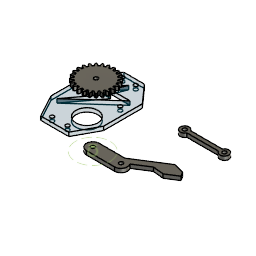
ARM (Autodesk Fusion 360 archive; units mm, degrees)
design "Untitled"
part number: 2026-04-05-15-25-42-375
Autodesk Fusion 360 part; units mm, degrees
note: some values were not read from the file. Chosen so that the rebuilt part matches the saved one: that a step has no effect. Set by a fixed rule: which sketch regions a step uses.
sketch "Sketch1" plane through (0, 0, 0) normal (0, 0, 1) x (1, 0, 0)
  line L0 (0, -5) -> (22, -5)
  arc A0 (22, -5) -> (22, 5) centre (22, 0) ccw
  line L1 (22, 5) -> (0, 5)
  arc A1 (0, 5) -> (0, -5) centre (0, 0) ccw
  line L2 (0, 0) -> (22, 0) construction
  line L3 (20.05, 5) -> (48.773, 23.1931)
  line L4 (48.773, 23.1931) -> (56.2338, 11.4141)
  line L5 (25.5276, -3.5434) -> (54.2034, 14.6197)
  line L6 (44.0321, 20.1901) -> (52.5034, 17.9377)
  line L7 (45.5663, 9.149) -> (37.2965, 10.0791)
  line L8 (37.2965, 10.0791) -> (26.0383, 2.9482)
  circle A2 centre (0, 0) radius 1.5
  circle A3 centre (22, 0) radius 1.5
  dimension "d1" = 22
  dimension "d2" = 5
  dimension "d3" = 147.65
  dimension "d4" = 34
  dimension "d6" = 1.95
  dimension "d7" = 3
  dimension "d8" = 3
  constraint tangent L0 A0
  constraint tangent A0 L1
  constraint parallel L0 L1
  constraint tangent L1 A1
  constraint tangent L0 A1
  constraint horizontal L2
  constraint coincident A1.centre L2.start
  constraint coincident L1 L3.start
  constraint perpendicular L3 L4
  constraint coincident A0 L5.start
  constraint coincident L4 L5.end
  constraint perpendicular L4 L5
  constraint coincident L3 L6.start
  constraint coincident L5 L7.start
  constraint coincident A0 L8.end
  constraint parallel L5 L8
  constraint concentric A1 A2
  constraint concentric A0 A3
  measures "d1" distance of A1.centre A0.centre
  measures "d2" radius of A1
  measures "d3" angle of L1 L3
  measures "d4" distance of L3.start L3.end
  measures "d6" horizontal distance of A0.centre L3.start
  measures "d7" diameter of A2
  measures "d8" diameter of A3
extrude "Extrude1" add sketch "Sketch1" along normal blind 3 contours L0 A0 L1 A1 | A0 L1 L3 L4 L5 L6 L7 L8 makes body 1
sketch "Sketch2" plane through (0, 0, 0) normal (0, 1, 0) x (1, 0, 0)
sketch "Sketch3" plane through (0, 0, 0) normal (0, 0, 1) x (1, 0, 0)
  circle A0 centre (24.0522, 47.6505) radius 3.5
  circle A1 centre (24.0522, 47.6505) radius 1.5
  circle A2 centre (55.0522, 47.6505) radius 3.5
  circle A3 centre (55.0522, 47.6505) radius 1.5
  line L0 (24.0522, 47.6505) -> (55.0522, 47.6505)
  line L1 (27.2144, 49.1505) -> (51.8899, 49.1505)
  line L2 (27.2144, 46.1505) -> (51.8899, 46.1505)
  dimension "d11" = 3
  dimension "d12" = 7
  dimension "d13" = 3
  dimension "d14" = 7
  dimension "d15" = 31
  dimension "d16" = 1.5
  constraint concentric A0 A1
  constraint concentric A2 A3
  constraint coincident A0.centre A1.centre
  constraint coincident A2.centre A3.centre
  constraint horizontal L0
  constraint coincident A0 L1.start
  constraint coincident A2 L1.end
  constraint horizontal L1
  constraint symmetric L0 L1.start L2.start
  constraint symmetric L0 L1.end L2.end
  measures "d11" diameter of A1
  measures "d12" diameter of A0
  measures "d13" diameter of A3
  measures "d14" diameter of A2
  measures "d15" distance of A0.centre A2.centre
  measures "d16" distance of L0 L1
extrude "Extrude2" add sketch "Sketch3" along normal blind 3 separate body makes body 2
sketch "Sketch4" plane through (0, 0, 0) normal (0, 0, 1) x (1, 0, 0)
  line L0 (0, 0) -> (0, 62)
  line L1 (0, 62) -> (-7.9898, 62)
  line L2 (-7.9898, 62) -> (-20.5, 47.8997)
  line L3 (-20.5, 17.5997) -> (-11, 0)
  line L4 (-11, 0) -> (0, 0)
  circle A0 centre (-6, 4) radius 1.5
  circle A1 centre (-13.5, 37.5997) radius 1.5
  circle A2 centre (-5.2398, 58) radius 1.5
  line L5 (-20.5, 47.8997) -> (-20.5, 17.5997)
  line L6 (20.5, 47.8997) -> (20.5, 17.5997)
  line L7 (7.9898, 62) -> (20.5, 47.8997)
  line L8 (20.5, 17.5997) -> (11, 0)
  line L9 (11, 0) -> (0, 0)
  line L10 (0, 0) -> (0, 62)
  circle A3 centre (5.2398, 58) radius 1.5
  circle A4 centre (6, 4) radius 1.5
  line L11 (0, 62) -> (7.9898, 62)
  circle A5 centre (13.5, 37.5997) radius 1.5
  circle A6 centre (7.5, 17.5997) radius 8.5
  line L12 (20.5, 17.5997) -> (0, 17.5997)
  dimension "d19" = 62
  dimension "d21" = 11
  dimension "d22" = 20
  dimension "d23" = 18.85
  dimension "d24" = 3
  dimension "d25" = 3
  dimension "d27" = 3
  dimension "d29" = 30.3
  dimension "d30" = 4
  dimension "d31" = 2.75
  dimension "d32" = 10.3
  dimension "d33" = 7
  dimension "d34" = 6
  dimension "d35" = 4
  dimension "d36" = 20.5
  dimension "d37" = 17
  dimension "d38" = 13
  constraint coincident L0.start L4.end
  constraint vertical L0
  constraint perpendicular L0 L1
  constraint perpendicular L0 L4
  constraint vertical L5
  constraint symmetric L4.end L0 L9.end
  constraint symmetric L1.start L0 L10.end
  constraint symmetric L0 L1.end L7.start
  constraint symmetric L0 L2.end L6.start
  constraint symmetric L0 L3.start L6.end
  constraint symmetric L0 L3.end L8.end
  constraint symmetric L0 L4.end L9.end
  constraint symmetric L0 A0 A4
  constraint symmetric L0 A1 A5
  constraint symmetric L0 A2 A3
  constraint coincident L10 L12.end
  constraint perpendicular L10 L12
  measures "d19" distance of L0.start L0.end
  measures "d21" distance of L3.end L0.start
  measures "d22" distance of L3.start L3.end
  measures "d23" distance of L1.end L2.end
  measures "d24" diameter of A0
  measures "d25" diameter of A1
  measures "d27" diameter of A2
  measures "d29" distance of L2.end L3.start
  measures "d30" distance of L1 A2.centre
  measures "d31" horizontal distance of L1.end A2.centre
  measures "d32" vertical distance of L2.end A1.centre
  measures "d33" distance of A1.centre L5
  measures "d34" distance of L0 A0.centre
  measures "d35" distance of L4 A0.centre
  measures "d36" distance of L0 L5
  measures "d37" diameter of A6
  measures "d38" distance of L6 A6.centre
extrude "Extrude3" add sketch "Sketch4" along normal blind 3 separate body contours L0 L1 L2 L3 L4 L5 L10 A6 | L0 L8 L9 L10 A6 L12 | L0 L6 L7 L10 L11 A6 L12 makes body 3
move_body "Move1" bodies 3 to x (1, 0, 0) y (0, 1, 0) z (0, 0, 1) at (0, 0, 2)
move_body "Move2" bodies 3 to x (1, 0, 0) y (0, 1, 0) z (0, 0, 1) at (-29.7095, 0, -1.4025)
sketch "Sketch5" plane through (0, 0, 3.5975) normal (0, 0, 1) x (-1, 0, 0)
  circle A0 centre (16.2095, -37.5997) radius 1.5
  circle A1 centre (43.2095, -37.5997) radius 1.5
  circle A2 centre (35.7095, -4) radius 1.5
  circle A3 centre (22.2095, -17.5997) radius 8.5
  circle A4 centre (24.4697, -58) radius 1.5
  circle A5 centre (23.7095, -4) radius 1.5
  circle A6 centre (34.9493, -58) radius 1.5
  line L0 (37.6993, -62) -> (50.2095, -47.8997)
  line L1 (50.2095, -47.8997) -> (50.2095, -17.5997)
  line L2 (50.2095, -17.5997) -> (40.7095, 0)
  line L3 (40.7095, 0) -> (18.7095, 0)
  line L4 (18.7095, 0) -> (9.2095, -17.5997)
  line L5 (9.2095, -17.5997) -> (9.2095, -47.8997)
  line L6 (9.2095, -47.8997) -> (21.7197, -62)
  line L7 (21.7197, -62) -> (37.6993, -62)
  line L8 (27, -55) -> (38, -42)
  line L9 (38, -42) -> (28, -42)
  line L10 (46, -18) -> (16, -45)
  line L11 (16, -45) -> (31, -45)
  line L12 (31, -45) -> (27, -55)
  line L13 (28, -42) -> (46, -18)
  constraint horizontal L9
  constraint parallel L9 L11
extrude "Extrude4" cut sketch "Sketch5" against normal blind 1 contours L8 L9 L10 L11 L12 L13 bodies 3
extrude "Extrude5" cut 1 faces at (-30, 35, 2.5975) along direction (0, 0, -1) blind 2 on bodies 3 bodies 3
sketch "Sketch6" plane through (0, 0, 0) normal (0, 0, 1) x (1, 0, 0)
sketch "Base Circle" plane through (0, 0, 0) normal (0, 0, 1) x (1, 0, 0)
  circle A0 centre (0, 0) radius 12.1984
  circle A1 centre (0, 0) radius 1.5
extrude "Extrude6" add sketch "Base Circle" along normal blind 3 separate body makes body 4
sketch "Gear Tooth" plane through (0, 0, 0) normal (0, 0, 1) x (1, 0, 0)
  spline S0 degree 5 poles (12.6449, -1.0183) (12.6506, -1.0187) (12.6618, -1.0195) (12.6788, -1.0202) (12.7014, -1.0204) (12.7297, -1.0195) (12.758, -1.0178) (12.7864, -1.0156) (12.8147, -1.0131) (12.8431, -1.0105) (12.8715, -1.0076) (12.8999, -1.0045) (12.9284, -1.0011) (12.9568, -0.9973) (12.9852, -0.9932) (13.0137, -0.9886) (13.0421, -0.9838) (13.0705, -0.9787) (13.099, -0.9733) (13.1274, -0.9678) (13.1559, -0.962) (13.1843, -0.956) (13.2127, -0.9498) (13.2412, -0.9433) (13.2696, -0.9366) (13.298, -0.9297) (13.3264, -0.9226) (13.3549, -0.9152) (13.3833, -0.9076) (13.4117, -0.8999) (13.4401, -0.8919) (13.4684, -0.8838) (13.4968, -0.8754) (13.5252, -0.8669) (13.5535, -0.8581) (13.5819, -0.8492) (13.6102, -0.8401) (13.6385, -0.8308) (13.6669, -0.8214) (13.6952, -0.8117) (13.7234, -0.8019) (13.7517, -0.7919) (13.78, -0.7817) (13.8082, -0.7714) (13.8365, -0.7609) (13.8647, -0.7502) (13.8929, -0.7393) (13.9211, -0.7283) (13.9492, -0.7171) (13.9774, -0.7058) (14.0055, -0.6943) (14.0337, -0.6826) (14.0618, -0.6708) (14.0898, -0.6588) (14.1179, -0.6467) (14.146, -0.6344) (14.174, -0.6219) (14.202, -0.6093) (14.23, -0.5966) (14.2579, -0.5837) (14.2859, -0.5706) (14.3138, -0.5574) (14.3417, -0.544) (14.3696, -0.5305) (14.3975, -0.5169) (14.4253, -0.5031) (14.4531, -0.4891) (14.4809, -0.4751) (14.5087, -0.4608) (14.5364, -0.4465) (14.5641, -0.4319) (14.5863, -0.4202) (14.6029, -0.4114) (14.6139, -0.4054) (14.6195, -0.4024) knots 0 0 0 0 0 0 0.01428571 0.02857143 0.04285714 0.05714286 0.07142857 0.08571429 0.1 0.11428571 0.12857143 0.14285714 0.15714286 0.17142857 0.18571429 0.2 0.21428571 0.22857143 0.24285714 0.25714286 0.27142857 0.28571429 0.3 0.31428571 0.32857143 0.34285714 0.35714286 0.37142857 0.38571429 0.4 0.41428571 0.42857143 0.44285714 0.45714286 0.47142857 0.48571429 0.5 0.51428571 0.52857143 0.54285714 0.55714286 0.57142857 0.58571429 0.6 0.61428571 0.62857143 0.64285714 0.65714286 0.67142857 0.68571429 0.7 0.71428571 0.72857143 0.74285714 0.75714286 0.77142857 0.78571429 0.8 0.81428571 0.82857143 0.84285714 0.85714286 0.87142857 0.88571429 0.9 0.91428571 0.92857143 0.94285714 0.95714286 0.97142857 0.98571429 1 1 1 1 1 1
  spline S1 degree 5 poles (12.6449, 1.0183) (12.6506, 1.0187) (12.6618, 1.0195) (12.6788, 1.0202) (12.7014, 1.0204) (12.7297, 1.0195) (12.758, 1.0178) (12.7864, 1.0156) (12.8147, 1.0131) (12.8431, 1.0105) (12.8715, 1.0076) (12.8999, 1.0045) (12.9284, 1.0011) (12.9568, 0.9973) (12.9852, 0.9932) (13.0137, 0.9886) (13.0421, 0.9838) (13.0705, 0.9787) (13.099, 0.9733) (13.1274, 0.9678) (13.1559, 0.962) (13.1843, 0.956) (13.2127, 0.9498) (13.2412, 0.9433) (13.2696, 0.9366) (13.298, 0.9297) (13.3264, 0.9226) (13.3549, 0.9152) (13.3833, 0.9076) (13.4117, 0.8999) (13.4401, 0.8919) (13.4684, 0.8838) (13.4968, 0.8754) (13.5252, 0.8669) (13.5535, 0.8581) (13.5819, 0.8492) (13.6102, 0.8401) (13.6385, 0.8308) (13.6669, 0.8214) (13.6952, 0.8117) (13.7234, 0.8019) (13.7517, 0.7919) (13.78, 0.7817) (13.8082, 0.7714) (13.8365, 0.7609) (13.8647, 0.7502) (13.8929, 0.7393) (13.9211, 0.7283) (13.9492, 0.7171) (13.9774, 0.7058) (14.0055, 0.6943) (14.0337, 0.6826) (14.0618, 0.6708) (14.0898, 0.6588) (14.1179, 0.6467) (14.146, 0.6344) (14.174, 0.6219) (14.202, 0.6093) (14.23, 0.5966) (14.2579, 0.5837) (14.2859, 0.5706) (14.3138, 0.5574) (14.3417, 0.544) (14.3696, 0.5305) (14.3975, 0.5169) (14.4253, 0.5031) (14.4531, 0.4891) (14.4809, 0.4751) (14.5087, 0.4608) (14.5364, 0.4465) (14.5641, 0.4319) (14.5863, 0.4202) (14.6029, 0.4114) (14.6139, 0.4054) (14.6195, 0.4024) knots 0 0 0 0 0 0 0.01428571 0.02857143 0.04285714 0.05714286 0.07142857 0.08571429 0.1 0.11428571 0.12857143 0.14285714 0.15714286 0.17142857 0.18571429 0.2 0.21428571 0.22857143 0.24285714 0.25714286 0.27142857 0.28571429 0.3 0.31428571 0.32857143 0.34285714 0.35714286 0.37142857 0.38571429 0.4 0.41428571 0.42857143 0.44285714 0.45714286 0.47142857 0.48571429 0.5 0.51428571 0.52857143 0.54285714 0.55714286 0.57142857 0.58571429 0.6 0.61428571 0.62857143 0.64285714 0.65714286 0.67142857 0.68571429 0.7 0.71428571 0.72857143 0.74285714 0.75714286 0.77142857 0.78571429 0.8 0.81428571 0.82857143 0.84285714 0.85714286 0.87142857 0.88571429 0.9 0.91428571 0.92857143 0.94285714 0.95714286 0.97142857 0.98571429 1 1 1 1 1 1
  arc A0 (14.6195, -0.4024) -> (14.6195, 0.4024) centre (0, 0) ccw
  line L0 (12.149, -0.9783) -> (12.6449, -1.0183)
  line L1 (12.149, 0.9783) -> (12.6449, 1.0183)
  line L2 (12.149, -0.9783) -> (12.149, 0.9783)
  point P0 (12.7841, -1.0157)
  point P1 (12.9241, -1.0016)
  point P2 (13.0647, -0.9797)
  point P3 (13.2057, -0.9513)
  point P4 (13.3469, -0.9172)
  point P5 (13.4884, -0.8779)
  point P6 (13.63, -0.8336)
  point P7 (13.7716, -0.7847)
  point P8 (13.9132, -0.7313)
  point P9 (14.0548, -0.6737)
  point P10 (14.1963, -0.6119)
  point P11 (14.3376, -0.546)
  point P12 (14.4787, -0.4761)
  point P13 (12.7841, 1.0157)
  point P14 (12.9241, 1.0016)
  point P15 (13.0647, 0.9797)
  point P16 (13.2057, 0.9513)
  point P17 (13.3469, 0.9172)
  point P18 (13.4884, 0.8779)
  point P19 (13.63, 0.8336)
  point P20 (13.7716, 0.7847)
  point P21 (13.9132, 0.7313)
  point P22 (14.0548, 0.6737)
  point P23 (14.1963, 0.6119)
  point P24 (14.3376, 0.546)
  point P25 (14.4787, 0.4761)
extrude "Extrude7" add sketch "Gear Tooth" along normal blind 3 bodies 4
fillet "Fillet1" radius 0.1 2 edges at (12.159, -0.9791, 1.5) (12.159, 0.9791, 1.5) on bodies 4
pattern_circular "C-Pattern1" count 24 over 360 about axis through (0, 0, 0) along (0, 0, 1) of "Extrude7", "Fillet1"
sketch "Diametrial Pitch Circle" plane through (0, 0, 0) normal (0, 0, 1) x (1, 0, 0)
  circle A0 centre (0, 0) radius 13.5 construction
move_body "Move3" bodies 4 to x (1, 0, 0) y (0, 1, 0) z (0, 0, 1) at (-51.4873, 13.4875, -38.6496)
move_body "Move4" bodies 4 to x (1, 0, 0) y (0, 1, 0) z (0, 0, 1) at (0, 24.1107, 24)
move_body "Move5" bodies 4 to x (1, 0, 0) y (0, 1, 0) z (0, 0, 1) at (14, 1, 18)
move_body "Move6" bodies 4 to x (1, 0, 0) y (0, 1, 0) z (0, 0, 1) at (0, 1.467, 4.1958)
named bodies: "Spur Gear (24 teeth)"

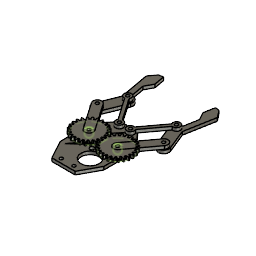
design "Untitled" references "Untitled"
part number: 2026-04-05-19-15-32-827
part number: 2026-04-05-19-18-36-866
description: Spur Gear; Module: 1.125; Num Teeth: 24; Pressure Angle: 20.0; Backlash: 0.00 mm
part number: 2026-04-05-19-21-24-649
part number: 2026-04-05-19-22-45-134
part number: 2026-04-05-19-22-48-026
part number: 2026-04-05-19-47-55-255
part number: 2026-04-06-19-05-38-398
Autodesk Fusion 360 part; units mm, degrees
other "Sketch1"
sketch "sketch 228" plane through (0, 0, 0) normal (0, 0, 1) x (1, 0, 0)
  line L0 (0, -5) -> (22, -5)
  arc A0 (22, -5) -> (22, 5) centre (22, 0) ccw
  line L1 (22, 5) -> (0, 5)
  arc A1 (0, 5) -> (0, -5) centre (0, 0) ccw
  line L2 (0, 0) -> (22, 0) construction
  line L3 (20.05, 5) -> (48.773, 23.1931)
  line L4 (48.773, 23.1931) -> (56.2338, 11.4141)
  line L5 (25.5276, -3.5434) -> (54.2034, 14.6197)
  line L6 (44.0321, 20.1901) -> (52.5034, 17.9377)
  line L7 (45.5663, 9.149) -> (37.2965, 10.0791)
  line L8 (37.2965, 10.0791) -> (26.0383, 2.9482)
  circle A2 centre (0, 0) radius 1.5
  circle A3 centre (22, 0) radius 1.5
extrude "Extrude1" add sketch "sketch 228" along normal blind 3 contours L0 A0 L1 A1 | A0 L1 L3 L4 L5 L6 L7 L8 makes body 1
copy_body "Body->Comp1" bodies 1 removing the originals makes body 2 in component "Component"
sketch "sketch 389" plane through (0, 0, 3.5975) normal (0, 0, 1) x (-1, 0, 0)
  circle A0 centre (16.2095, -37.5997) radius 1.5
  circle A1 centre (43.2095, -37.5997) radius 1.5
  circle A2 centre (35.7095, -4) radius 1.5
  circle A3 centre (22.2095, -17.5997) radius 8.5
  circle A4 centre (24.4697, -58) radius 1.5
  circle A5 centre (23.7095, -4) radius 1.5
  circle A6 centre (34.9493, -58) radius 1.5
  line L0 (37.6993, -62) -> (50.2095, -47.8997)
  line L1 (50.2095, -47.8997) -> (50.2095, -17.5997)
  line L2 (50.2095, -17.5997) -> (40.7095, 0)
  line L3 (40.7095, 0) -> (18.7095, 0)
  line L4 (18.7095, 0) -> (9.2095, -17.5997)
  line L5 (9.2095, -17.5997) -> (9.2095, -47.8997)
  line L6 (9.2095, -47.8997) -> (21.7197, -62)
  line L7 (21.7197, -62) -> (37.6993, -62)
  line L8 (27, -55) -> (38, -42)
  line L9 (38, -42) -> (28, -42)
  line L10 (46, -18) -> (16, -45)
  line L11 (16, -45) -> (31, -45)
  line L12 (31, -45) -> (27, -55)
  line L13 (28, -42) -> (46, -18)
extrude "Extrude2" add sketch "sketch 389" along normal blind 3 separate body makes body 3
sketch "Base Circle" plane through (0, 0, 0) normal (0, 0, 1) x (1, 0, 0) in component "Spur Gear 24 teeth"
  circle A0 centre (0, 0) radius 12.1984
  circle A1 centre (0, 0) radius 1.5
extrude "Extrude1'" add sketch "Base Circle" along normal blind 3 separate body makes body 4 in component "Spur Gear 24 teeth"
sketch "Gear Tooth" plane through (0, 0, 0) normal (0, 0, 1) x (1, 0, 0) in component "Spur Gear 24 teeth"
  spline S0 degree 5 poles (12.6449, -1.0183) (12.6506, -1.0187) (12.6618, -1.0195) (12.6788, -1.0202) (12.7014, -1.0204) (12.7297, -1.0195) (12.758, -1.0178) (12.7864, -1.0156) (12.8147, -1.0131) (12.8431, -1.0105) (12.8715, -1.0076) (12.8999, -1.0045) (12.9284, -1.0011) (12.9568, -0.9973) (12.9852, -0.9932) (13.0137, -0.9886) (13.0421, -0.9838) (13.0705, -0.9787) (13.099, -0.9733) (13.1274, -0.9678) (13.1559, -0.962) (13.1843, -0.956) (13.2127, -0.9498) (13.2412, -0.9433) (13.2696, -0.9366) (13.298, -0.9297) (13.3264, -0.9226) (13.3549, -0.9152) (13.3833, -0.9076) (13.4117, -0.8999) (13.4401, -0.8919) (13.4684, -0.8838) (13.4968, -0.8754) (13.5252, -0.8669) (13.5535, -0.8581) (13.5819, -0.8492) (13.6102, -0.8401) (13.6385, -0.8308) (13.6669, -0.8214) (13.6952, -0.8117) (13.7234, -0.8019) (13.7517, -0.7919) (13.78, -0.7817) (13.8082, -0.7714) (13.8365, -0.7609) (13.8647, -0.7502) (13.8929, -0.7393) (13.9211, -0.7283) (13.9492, -0.7171) (13.9774, -0.7058) (14.0055, -0.6943) (14.0337, -0.6826) (14.0618, -0.6708) (14.0898, -0.6588) (14.1179, -0.6467) (14.146, -0.6344) (14.174, -0.6219) (14.202, -0.6093) (14.23, -0.5966) (14.2579, -0.5837) (14.2859, -0.5706) (14.3138, -0.5574) (14.3417, -0.544) (14.3696, -0.5305) (14.3975, -0.5169) (14.4253, -0.5031) (14.4531, -0.4891) (14.4809, -0.4751) (14.5087, -0.4608) (14.5364, -0.4465) (14.5641, -0.4319) (14.5863, -0.4202) (14.6029, -0.4114) (14.6139, -0.4054) (14.6195, -0.4024) knots 0 0 0 0 0 0 0.01428571 0.02857143 0.04285714 0.05714286 0.07142857 0.08571429 0.1 0.11428571 0.12857143 0.14285714 0.15714286 0.17142857 0.18571429 0.2 0.21428571 0.22857143 0.24285714 0.25714286 0.27142857 0.28571429 0.3 0.31428571 0.32857143 0.34285714 0.35714286 0.37142857 0.38571429 0.4 0.41428571 0.42857143 0.44285714 0.45714286 0.47142857 0.48571429 0.5 0.51428571 0.52857143 0.54285714 0.55714286 0.57142857 0.58571429 0.6 0.61428571 0.62857143 0.64285714 0.65714286 0.67142857 0.68571429 0.7 0.71428571 0.72857143 0.74285714 0.75714286 0.77142857 0.78571429 0.8 0.81428571 0.82857143 0.84285714 0.85714286 0.87142857 0.88571429 0.9 0.91428571 0.92857143 0.94285714 0.95714286 0.97142857 0.98571429 1 1 1 1 1 1
  spline S1 degree 5 poles (12.6449, 1.0183) (12.6506, 1.0187) (12.6618, 1.0195) (12.6788, 1.0202) (12.7014, 1.0204) (12.7297, 1.0195) (12.758, 1.0178) (12.7864, 1.0156) (12.8147, 1.0131) (12.8431, 1.0105) (12.8715, 1.0076) (12.8999, 1.0045) (12.9284, 1.0011) (12.9568, 0.9973) (12.9852, 0.9932) (13.0137, 0.9886) (13.0421, 0.9838) (13.0705, 0.9787) (13.099, 0.9733) (13.1274, 0.9678) (13.1559, 0.962) (13.1843, 0.956) (13.2127, 0.9498) (13.2412, 0.9433) (13.2696, 0.9366) (13.298, 0.9297) (13.3264, 0.9226) (13.3549, 0.9152) (13.3833, 0.9076) (13.4117, 0.8999) (13.4401, 0.8919) (13.4684, 0.8838) (13.4968, 0.8754) (13.5252, 0.8669) (13.5535, 0.8581) (13.5819, 0.8492) (13.6102, 0.8401) (13.6385, 0.8308) (13.6669, 0.8214) (13.6952, 0.8117) (13.7234, 0.8019) (13.7517, 0.7919) (13.78, 0.7817) (13.8082, 0.7714) (13.8365, 0.7609) (13.8647, 0.7502) (13.8929, 0.7393) (13.9211, 0.7283) (13.9492, 0.7171) (13.9774, 0.7058) (14.0055, 0.6943) (14.0337, 0.6826) (14.0618, 0.6708) (14.0898, 0.6588) (14.1179, 0.6467) (14.146, 0.6344) (14.174, 0.6219) (14.202, 0.6093) (14.23, 0.5966) (14.2579, 0.5837) (14.2859, 0.5706) (14.3138, 0.5574) (14.3417, 0.544) (14.3696, 0.5305) (14.3975, 0.5169) (14.4253, 0.5031) (14.4531, 0.4891) (14.4809, 0.4751) (14.5087, 0.4608) (14.5364, 0.4465) (14.5641, 0.4319) (14.5863, 0.4202) (14.6029, 0.4114) (14.6139, 0.4054) (14.6195, 0.4024) knots 0 0 0 0 0 0 0.01428571 0.02857143 0.04285714 0.05714286 0.07142857 0.08571429 0.1 0.11428571 0.12857143 0.14285714 0.15714286 0.17142857 0.18571429 0.2 0.21428571 0.22857143 0.24285714 0.25714286 0.27142857 0.28571429 0.3 0.31428571 0.32857143 0.34285714 0.35714286 0.37142857 0.38571429 0.4 0.41428571 0.42857143 0.44285714 0.45714286 0.47142857 0.48571429 0.5 0.51428571 0.52857143 0.54285714 0.55714286 0.57142857 0.58571429 0.6 0.61428571 0.62857143 0.64285714 0.65714286 0.67142857 0.68571429 0.7 0.71428571 0.72857143 0.74285714 0.75714286 0.77142857 0.78571429 0.8 0.81428571 0.82857143 0.84285714 0.85714286 0.87142857 0.88571429 0.9 0.91428571 0.92857143 0.94285714 0.95714286 0.97142857 0.98571429 1 1 1 1 1 1
  arc A0 (14.6195, -0.4024) -> (14.6195, 0.4024) centre (0, 0) ccw
  line L0 (12.149, -0.9783) -> (12.6449, -1.0183)
  line L1 (12.149, 0.9783) -> (12.6449, 1.0183)
  line L2 (12.149, -0.9783) -> (12.149, 0.9783)
  point P0 (12.7841, -1.0157)
  point P1 (12.9241, -1.0016)
  point P2 (13.0647, -0.9797)
  point P3 (13.2057, -0.9513)
  point P4 (13.3469, -0.9172)
  point P5 (13.4884, -0.8779)
  point P6 (13.63, -0.8336)
  point P7 (13.7716, -0.7847)
  point P8 (13.9132, -0.7313)
  point P9 (14.0548, -0.6737)
  point P10 (14.1963, -0.6119)
  point P11 (14.3376, -0.546)
  point P12 (14.4787, -0.4761)
  point P13 (12.7841, 1.0157)
  point P14 (12.9241, 1.0016)
  point P15 (13.0647, 0.9797)
  point P16 (13.2057, 0.9513)
  point P17 (13.3469, 0.9172)
  point P18 (13.4884, 0.8779)
  point P19 (13.63, 0.8336)
  point P20 (13.7716, 0.7847)
  point P21 (13.9132, 0.7313)
  point P22 (14.0548, 0.6737)
  point P23 (14.1963, 0.6119)
  point P24 (14.3376, 0.546)
  point P25 (14.4787, 0.4761)
extrude "Extrude2'" add sketch "Gear Tooth" along normal blind 3 bodies 4 in component "Spur Gear 24 teeth"
fillet "Fillet1" radius 0.1 2 edges at (12.159, -0.9791, 1.5) (12.159, 0.9791, 1.5) on bodies 4 in component "Spur Gear 24 teeth"
pattern_circular "C-Pattern1" count 24 over 360 about axis through (0, 0, 0) along (0, 0, 1) of "Extrude2'", "Fillet1" in component "Spur Gear 24 teeth"
sketch "Diametrial Pitch Circle" plane through (0, 0, 0) normal (0, 0, 1) x (1, 0, 0) in component "Spur Gear 24 teeth"
  circle A0 centre (0, 0) radius 13.5 construction
sketch "sketch 288" plane through (0, 0, 0) normal (0, 0, 1) x (1, 0, 0)
  circle A0 centre (24.0522, 47.6505) radius 3.5
  circle A1 centre (24.0522, 47.6505) radius 1.5
  circle A2 centre (55.0522, 47.6505) radius 3.5
  circle A3 centre (55.0522, 47.6505) radius 1.5
  line L0 (24.0522, 47.6505) -> (55.0522, 47.6505)
  line L1 (27.2144, 49.1505) -> (51.8899, 49.1505)
  line L2 (27.2144, 46.1505) -> (51.8899, 46.1505)
extrude "Extrude3" add sketch "sketch 288" along normal blind 3 separate body makes body 5
copy_body "Body->Comp2" bodies 3 removing the originals makes body 6 in component "Component'"
copy_body "Body->Comp3" bodies 5 removing the originals makes body 7 in component "Component''"
move_body "Move1" bodies 2 to x (1, 0, 0) y (0, 1, 0) z (0, 0, 1) at (33, 0, 16) in component "Component"
move_face "MoveFace1" by (-0.3743, 2.096, 0) 1 faces at (8.6004, 0, 3) on bodies 4 in component "Spur Gear 24 teeth"
form "Form1" [no effect]
form "Form2" [no effect]
sketch "Sketch1" plane through (0, 0, 0) normal (1, 0, 0) x (0, 1, 0)
  circle A0 centre (21, 3) radius 7.8102
sketch "Sketch2" plane through (0, 0, 0) normal (0, 0, 1) x (1, 0, 0)
  line L0 (19.74, -20.4) -> (19.74, 10.6)
  arc A0 (19.74, 10.6) -> (11.74, 10.6) centre (15.74, 10.6) ccw
  line L1 (11.74, 10.6) -> (11.74, -20.4)
  arc A1 (11.74, -20.4) -> (19.74, -20.4) centre (15.74, -20.4) ccw
  line L2 (15.74, -20.4) -> (15.74, 10.6) construction
  circle A2 centre (15.74, 10.6) radius 1.5
  circle A3 centre (15.74, -20.4) radius 1.5
  dimension "d51" = 31
  dimension "d52" = 8
  dimension "d53" = 3
  dimension "d54" = 3
  constraint tangent L0 A0
  constraint tangent A0 L1
  constraint parallel L0 L1
  constraint tangent L1 A1
  constraint tangent L0 A1
  constraint vertical L2
  constraint concentric A0 A2
  constraint concentric A1 A3
  measures "d51" distance of A1.centre A0.centre
  measures "d52" diameter of A0
  measures "d53" diameter of A2
  measures "d54" diameter of A3
extrude "Extrude5" add sketch "Sketch2" along normal blind 3 separate body makes body 8
copy_body "Body->Comp5" bodies 8 removing the originals makes body 9 in component "Component''''"
ref_plane "WorkPlane1" through (-29.7095, 32.7497, 5.0975) normal (-1, 0, 0) x (0, -1, 0)
mirror "MirrorComponent1" about plane through (0, 0, 0) normal (0, 0, 1) of bodies 2 makes body 10 in component "Component1(Mirror)"
mirror "MirrorComponent1'" about plane through (0, 0, 0) normal (0, 0, 1) of bodies 7 makes body 11 in component "Component4(Mirror)"
hole "Hole1" at (-29.6439, 26.91, 3.5975) direction (0, 0, 1) diameter 4 depth 30 tip angle 118 bodies 6 in component "Component'"
component "Spur Gear 24 teeth" placed x (0.822159, 0.569258, 0) y (-0.569258, 0.822159, 0) z (0, 0, 1) at (-43.2095, 37.5997, 6.5975)
component "Component''" placed x (-0.569547, 0.821958, 0) y (-0.821958, -0.569547, 0) z (0, 0, 1) at (17.9163, 65.3693, 6.5975)
component "Component'" placed x (1, 0, 0) y (0, 1, 0) z (0, 0, 1) at (0, 0, 0)
component "Spur Gear 24 teeth" placed x (0.731354, -0.681998, 0) y (0.681998, 0.731354, 0) z (0, 0, 1) at (-16.2095, 37.5997, 6.5975)
component "Component'''" placed x (1, 0, 0) y (0, 1, 0) z (0, 0, 1) at (0, 0, 0)
component "Component''''" placed x (0.822159, 0.569258, 0) y (-0.569258, 0.822159, 0) z (0, 0, 1) at (-67.7631, 45.4116, 6.5975)
component "Component''''" placed x (0.803857, -0.594823, 0) y (0.594823, 0.803857, 0) z (0, 0, 1) at (-16.7278, 63.3609, 6.5975)
component "Component" placed x (0.375054, 0.927003, 0) y (-0.927003, 0.375054, 0) z (0, 0, 1) at (-73.2333, 32.4956, -12.4025)
component "Component4(Mirror)" placed x (0.5951, 0.803651, 0) y (0.803651, -0.5951, 0) z (0, 0, -1) at (-77.0775, 67.0273, 6.5975)
component "Component1(Mirror)" placed x (-0.375071, 0.926996, 0) y (0.926996, 0.375071, 0) z (0, 0, -1) at (14.6074, 31.9284, -12.4025)
